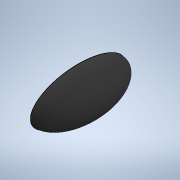
# Autodesk Inventor part: SW-S01
Saved by Autodesk Inventor 2022 (Build 260153000, 153)
## iProperties
Company: El Camino College
Created: 2023-04-07
Part Number: SW-S01
Material: Rubber, Silicone
Document SubType Name: Modeling
Designer: Edgar Tejada
Density: 1.25 g/cm^3
Appearance: Rubber - Black
Mass: 81.8123 g
Surface Area: 106.39 cm^2
Volume: 65.4498 cm^3
Project: Egonomic Fight Stick
Author: Edgar Tejada
Title: Silicone Wrist Support
Subject: Ergonomic Fight Stick
Autodesk Inventor part; units mm, degrees
ref_plane "YZ Plane" through (0, 0, 0) normal (1, 0, 0) x (0, 1, 0)
ref_plane "XZ Plane" through (0, 0, 0) normal (0, 1, 0) x (-1, 0, 0)
ref_plane "XY Plane" through (0, 0, 0) normal (0, 0, 1) x (1, 0, 0)
sketch "Sketch1" plane through (0, 0, 0) normal (1, 0, 0) x (0, 1, 0)
  line L0 (0, 50) -> (0, -50)
  ellipse E0 centre (0, 0) end of major axis (0, -50) minor radius 25
  line L1 (0, -70) -> (0, 70) construction
  dimension "d5" = 50
  dimension "d6" = 25
  dimension "d0" = 50
  dimension "d1" = 50
  constraints: 2 end point, 2 vertical, 2 vertical alignment, 1 coincident, 3 other
  measures "d0" distance of L0.end point (0, 0)
  measures "d1" distance of L0.start point (0, 0)
revolve "Revolution1" add sketch "Sketch1" angle 180 about axis through (0, 0, -10) along (0, 0, -1) picked at (8.2995, 1.4995) contours E0 L0
equation "\"d1\" = d0"
body "Solid1"
